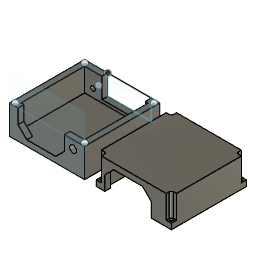
lötdampfabzug_ (Autodesk Fusion 360 design; units mm, degrees)
part number: 2026-02-08-19-36-14-347
Autodesk Fusion 360 part; units mm, degrees
sketch "Skizze1" plane through (0, 0, 0) normal (0, 0, 1) x (1, 0, 0)
  line L0 (0, 0) -> (130, 0)
  line L1 (130, 0) -> (130, 130)
  line L2 (130, 130) -> (0, 130)
  line L3 (0, 130) -> (0, 0)
  dimension "d1" = 130
  dimension "d2" = 130
  constraint horizontal L0
  constraint vertical L1
  constraint horizontal L2
  constraint vertical L3
  constraint coincident L0.start L3.end
  measures "d1" distance of L0.start L0.end
  measures "d2" distance of L0.start L2.end
extrude "Extrusion1" add sketch "Skizze1" along normal blind 100 makes body 1
shell "Schale1" thickness 10 removed faces 0 bodies 1
ref_plane "Arbeitsebene2" through (65, 65, 50) normal (0, 0, 1) x (1, 0, 0)
split "Teilen1" by plane through (65, 65, 50) normal (0, 0, 1) bodies 1 makes body 2 at (43.3333, 86.6667, 100)
sketch "Skizze3" plane through (0, 0, 50) normal (0, 0, 1) x (1, 0, 0)
  circle A0 centre (5, 125) radius 2.25
  circle A1 centre (5, 5) radius 2.25
  circle A2 centre (125, 125) radius 2.25
  circle A3 centre (125, 5) radius 2.25
  dimension "d20" = 4.5
  measures "d20" diameter of A0
extrude "Extrusion4" cut sketch "Skizze3" against normal blind 15 contours A0 | A1 bodies 1
sketch "Skizze4" plane through (0, 0, 0) normal (0, -1, 0) x (1, 0, 0)
  line L0 (0, 50) -> (130, 50)
  line L1 (130, 50) -> (130, 100)
  line L2 (130, 100) -> (0, 100)
  line L3 (0, 100) -> (0, 50)
sketch "Skizze5" plane through (0, 0, 0) normal (0, -1, 0) x (1, 0, 0)
  line L0 (130, 50) -> (0, 50)
  line L1 (0, 50) -> (0, 0)
  line L2 (0, 0) -> (130, 0)
  line L3 (130, 0) -> (130, 50)
sketch "Skizze6" plane through (0, 0, 0) normal (0, -1, 0) x (1, 0, 0)
  line L0 (95, 90) -> (80, 90)
  line L1 (95, 90) -> (95, 75)
  line L2 (95, 75) -> (80, 90)
  line L3 (95, 10) -> (80, 10)
  line L4 (95, 10) -> (95, 25)
  line L5 (95, 25) -> (80, 10)
  line L6 (15, 10) -> (30, 10)
  line L7 (15, 10) -> (15, 25)
  line L8 (15, 25) -> (30, 10)
  line L9 (15, 90) -> (15, 75)
  line L10 (15, 75) -> (30, 90)
  line L11 (30, 90) -> (15, 90)
  line L12 (95, 75) -> (95, 25)
  line L13 (80, 10) -> (30, 10)
  line L14 (15, 25) -> (15, 75)
  line L15 (30, 90) -> (80, 90)
  dimension "d29" = 15
  dimension "d30" = 15
  dimension "d31" = 15
  dimension "d32" = 15
  dimension "d33" = 15
  dimension "d34" = 15
  dimension "d37" = 15
  constraint horizontal L0
  constraint perpendicular L0 L1
  constraint perpendicular L1 L3
  constraint perpendicular L3 L4
  constraint perpendicular L4 L6
  constraint perpendicular L6 L7
  constraint perpendicular L6 L9
  constraint perpendicular L8 L10
  constraint perpendicular L9 L11
  constraint parallel L4 L12
  constraint perpendicular L12 L13
  constraint perpendicular L13 L14
  constraint perpendicular L14 L15
  measures "d29" distance of L0.start L0.end
  measures "d30" distance of L3.start L3.end
  measures "d31" distance of L3.start L4.end
  measures "d32" distance of L6.start L6.end
  measures "d33" distance of L6.start L7.end
  measures "d34" distance of L9.start L9.end
  measures "d37" distance of L0.start L1.end
extrude "Extrusion5" cut sketch "Skizze6" against normal blind 15 contours L2 L5 L8 L10 L12 L13 L14 L15 bodies 1 2
sketch "Skizze9" plane through (0, 0, 50) normal (0, 0, 1) x (-1, 0, 0)
  line L0 (-95, -10) -> (-95, 0)
  line L1 (-95, 0) -> (-130, 0)
  line L2 (-130, 0) -> (-130, -130)
  line L3 (-130, -130) -> (0, -130)
  line L4 (0, -130) -> (0, 0)
  line L5 (0, 0) -> (-15, 0)
  line L6 (-15, 0) -> (-15, -10)
  line L7 (-15, -10) -> (-10, -10)
  line L8 (-10, -10) -> (-10, -120)
  line L9 (-10, -120) -> (-120, -120)
  line L10 (-120, -120) -> (-120, -10)
  line L11 (-120, -10) -> (-95, -10)
  circle A0 centre (-5, -5) radius 2.25
  circle A1 centre (-5, -125) radius 2.25
extrude "Extrusion7" cut sketch "Skizze3" against normal blind 15 contours A2 | A3 bodies 1
sketch "Skizze11" plane through (0, 0, 100) normal (0, 0, 1) x (-1, 0, 0)
  line L0 (0, -130) -> (0, 0)
  line L1 (0, 0) -> (-130, 0)
  line L2 (-130, 0) -> (-130, -130)
  line L3 (-130, -130) -> (0, -130)
  line L4 (0, 0) -> (-9, 0)
  line L5 (-9, 0) -> (-9, -9)
  line L6 (-9, -9) -> (0, -9)
  line L7 (0, -9) -> (0, 0)
  line L8 (-130, 0) -> (-121, 0)
  line L9 (-121, 0) -> (-121, -9)
  line L10 (-121, -9) -> (-130, -9)
  line L11 (-130, -9) -> (-130, 0)
  line L12 (-130, -130) -> (-121, -130)
  line L13 (-121, -130) -> (-121, -121)
  line L14 (-121, -121) -> (-130, -121)
  line L15 (-130, -121) -> (-130, -130)
  line L16 (0, -130) -> (-9, -130)
  line L17 (-9, -130) -> (-9, -121)
  line L18 (-9, -121) -> (0, -121)
  line L19 (0, -121) -> (0, -130)
  dimension "d51" = 9
  dimension "d52" = 9
  dimension "d53" = 9
  dimension "d54" = 9
  dimension "d55" = 9
  dimension "d56" = 9
  dimension "d57" = 9
  dimension "d58" = 9
  constraint horizontal L4
  constraint vertical L5
  constraint horizontal L6
  constraint vertical L7
  constraint coincident L0.end L1.start
  constraint horizontal L8
  constraint vertical L9
  constraint horizontal L10
  constraint vertical L11
  constraint coincident L1.end L2.start
  constraint horizontal L12
  constraint vertical L13
  constraint horizontal L14
  constraint vertical L15
  constraint coincident L2.end L3.start
  constraint horizontal L16
  constraint vertical L17
  constraint horizontal L18
  constraint vertical L19
  constraint coincident L0.start L3.end
  measures "d51" distance of L5.end L6.end
  measures "d52" distance of L4.end L5.end
  measures "d53" distance of L1.end L8.end
  measures "d54" distance of L1.end L10.end
  measures "d55" distance of L2.end L12.end
  measures "d56" distance of L2.end L14.end
  measures "d57" distance of L0.start L16.end
  measures "d58" distance of L0.start L18.end
extrude "Extrusion8" cut sketch "Skizze11" against normal blind 40 contours L0 L3 L16 L17 L18 L19 | L0 L1 L4 L5 L6 L7 | L2 L3 L12 L13 L14 L15 | L1 L2 L8 L9 L10 L11 bodies 2
fillet "Abrundung1" radius 4 1 edges at (9, 121, 80) on bodies 2
fillet "Abrundung2" radius 4 3 edges at (121, 121, 80) (9, 9, 80) (121, 9, 80) on bodies 2
sketch "Skizze12" plane through (0, 0, 60) normal (0, 0, 1) x (-1, 0, 0)
  arc A0 (-125, -9) -> (-121, -5) centre (-125, -5) ccw
  line L0 (-121, -5) -> (-121, 0)
  line L1 (-121, 0) -> (-130, 0)
  line L2 (-130, 0) -> (-130, -9)
  line L3 (-130, -9) -> (-125, -9)
  circle A1 centre (-125, -5) radius 1.75
  dimension "d65" = 3.5
  constraint concentric A0 A1
  measures "d65" diameter of A1
extrude "Extrusion9" cut sketch "Skizze12" against normal blind 25 contours A1 bodies 2
sketch "Skizze13" plane through (0, 0, 60) normal (0, 0, 1) x (-1, 0, 0)
  circle A0 centre (-125, -5) radius 1.75
  arc A1 (-125, -9) -> (-121, -5) centre (-125, -5) ccw
  line L0 (-121, -5) -> (-121, 0)
  line L1 (-121, 0) -> (-130, 0)
  line L2 (-130, 0) -> (-130, -9)
  line L3 (-130, -9) -> (-125, -9)
  circle A2 centre (-125, -5) radius 2.5
  dimension "d68" = 5
  constraint concentric A0 A2
  measures "d68" diameter of A2
extrude "Extrusion10" cut sketch "Skizze13" against normal blind 3 contours A2 bodies 2
sketch "Skizze14" plane through (0, 0, 60) normal (0, 0, 1) x (-1, 0, 0)
  arc A0 (-121, -125) -> (-125, -121) centre (-125, -125) ccw
  line L0 (-125, -121) -> (-130, -121)
  line L1 (-130, -121) -> (-130, -130)
  line L2 (-130, -130) -> (-121, -130)
  line L3 (-121, -130) -> (-121, -125)
  circle A1 centre (-125, -125) radius 1.75
  dimension "d71" = 3.5
  constraint concentric A0 A1
  measures "d71" diameter of A1
extrude "Extrusion11" cut sketch "Skizze14" against normal blind 100 contours A1 bodies 2
sketch "Skizze15" plane through (0, 0, 60) normal (0, 0, 1) x (-1, 0, 0)
  circle A0 centre (-125, -125) radius 1.75
  arc A1 (-121, -125) -> (-125, -121) centre (-125, -125) ccw
  line L0 (-125, -121) -> (-130, -121)
  line L1 (-130, -121) -> (-130, -130)
  line L2 (-130, -130) -> (-121, -130)
  line L3 (-121, -130) -> (-121, -125)
  circle A2 centre (-125, -125) radius 2.5
  dimension "d74" = 5
  constraint concentric A0 A2
  measures "d74" diameter of A2
extrude "Extrusion12" cut sketch "Skizze15" against normal blind 3 contours A2 bodies 2
sketch "Skizze16" plane through (0, 0, 60) normal (0, 0, 1) x (-1, 0, 0)
  arc A0 (-5, -121) -> (-9, -125) centre (-5, -125) ccw
  line L0 (-9, -125) -> (-9, -130)
  line L1 (-9, -130) -> (0, -130)
  line L2 (0, -130) -> (0, -121)
  line L3 (0, -121) -> (-5, -121)
  circle A1 centre (-5, -125) radius 1.75
  dimension "d77" = 3.5
  constraint concentric A0 A1
  measures "d77" diameter of A1
extrude "Extrusion13" cut sketch "Skizze16" against normal blind 100 contours A1 bodies 2
sketch "Skizze17" plane through (0, 0, 60) normal (0, 0, 1) x (-1, 0, 0)
  circle A0 centre (-5, -125) radius 1.75
  arc A1 (-5, -121) -> (-9, -125) centre (-5, -125) ccw
  line L0 (-9, -125) -> (-9, -130)
  line L1 (-9, -130) -> (0, -130)
  line L2 (0, -130) -> (0, -121)
  line L3 (0, -121) -> (-5, -121)
  circle A2 centre (-5, -125) radius 2.5
  dimension "d80" = 5
  constraint concentric A0 A2
  measures "d80" diameter of A2
extrude "Extrusion14" cut sketch "Skizze17" against normal blind 3 contours A2 bodies 2
sketch "Skizze18" plane through (0, 0, 60) normal (0, 0, 1) x (-1, 0, 0)
  arc A0 (-9, -5) -> (-5, -9) centre (-5, -5) ccw
  line L0 (-5, -9) -> (0, -9)
  line L1 (0, -9) -> (0, 0)
  line L2 (0, 0) -> (-9, 0)
  line L3 (-9, 0) -> (-9, -5)
  circle A1 centre (-5, -5) radius 1.75
  dimension "d83" = 3.5
  constraint concentric A0 A1
  measures "d83" diameter of A1
extrude "Extrusion15" cut sketch "Skizze18" against normal blind 20 contours A1 bodies 2
sketch "Skizze19" plane through (0, 0, 60) normal (0, 0, 1) x (-1, 0, 0)
  circle A0 centre (-5, -5) radius 1.75
  arc A1 (-9, -5) -> (-5, -9) centre (-5, -5) ccw
  line L0 (-5, -9) -> (0, -9)
  line L1 (0, -9) -> (0, 0)
  line L2 (0, 0) -> (-9, 0)
  line L3 (-9, 0) -> (-9, -5)
  circle A2 centre (-5, -5) radius 2.5
  dimension "d86" = 5
  constraint concentric A0 A2
  measures "d86" diameter of A2
extrude "Extrusion16" cut sketch "Skizze19" against normal blind 3 contours A2 bodies 2
sketch "Skizze20" plane through (0, 0, 0) normal (0, -1, 0) x (1, 0, 0)
  circle A0 centre (110, 36) radius 6
  dimension "d90" = 12
  measures "d90" diameter of A0
extrude "Extrusion17" cut sketch "Skizze20" against normal blind 20 bodies 1
sketch "Skizze21" plane through (0, 0, 0) normal (0, -1, 0) x (1, 0, 0)
sketch "Skizze22" plane through (0, 130, 0) normal (0, 1, 0) x (-1, 0, 0)
  line L0 (0, 50) -> (-130, 50)
  line L1 (-130, 50) -> (-130, 0)
  line L2 (-130, 0) -> (0, 0)
  line L3 (0, 0) -> (0, 50)
  circle A0 centre (-24.4138, 23.7228) radius 4
  line L4 (-115, 15) -> (-40, 15)
  line L5 (-40, 15) -> (-40, 50)
  line L6 (-40, 50) -> (-115, 50)
  line L7 (-115, 50) -> (-115, 15)
  dimension "d97" = 8
  constraint horizontal L4
  constraint vertical L5
  constraint horizontal L6
  constraint vertical L7
  constraint coincident L0 L5.end
  measures "d97" diameter of A0
extrude "Extrusion18" cut sketch "Skizze22" against normal blind 40 contours A0 bodies 1
extrude "Extrusion19" cut sketch "Skizze22" against normal blind 20 contours L0 L4 L5 L6 L7 bodies 1
move_body "Verschieben1" bodies 2 to x (1, 0, 0) y (0, 1, 0) z (0, 0, 1) at (150, 0, -50)
